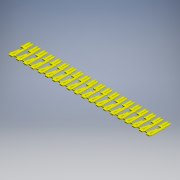
# Autodesk Inventor part: IDSD-20_pin
Saved by Autodesk Inventor 2017.3 (Build 213256000, 256)
## iProperties
Part Number: IDSD-20_pin
Material: Generic
Catalog Web Link: www.cadenas.de
Description: IDSS, IDSD Series - Pin-.100" Slim Body, IDC Ribbon Cable Assembly, Socket
Vendor: SAMTEC
Document SubType Name: Modeling
Designer: partserver
Manufacturer: SAMTEC
Mass: 0.0644285 g
Surface Area: 6.03509 cm^2
Volume: 0.0644285 cm^3
Density: 1 g/cm^3
Appearance: PSOLRGB-255-255-0
Category: PARTsolutions
Company: SAMTEC
Title: IDSD-20_pin
Author: Cadenas PARTsolutions
Comments: .100" Slim Body, IDC Ribbon Cable Assembly, Socket
PSOL_IDENT_0: {$CADENAS_DATA\23d-libs\samtec\modelling\idsd\parts\idsd_pin.prj},182 {VTYP=3D},{NB=IDSD-20_pin},{LI
PSOL_IDENT_1: NA=IDSD-20_pin},{NN=IDSS, IDSD Series - Pin},{DATE=12.08.2019 09:04:52},{GEOMDATE=04.12.2014 16:05:0
PSOL_IDENT_2: 0},{VERSION=},{LINEID=20},{WBVAR=POS},{WBNUMERIC=}  {NB=IDSD-20_pin},{LINA=IDSD-20_pin},{KT=DUMMY},{
PSOL_IDENT_3: PN=IDSD-20},{SERIES=IDSD},{POS=20},{POSNO=20},{A=2.05900000},{B=0.20},{C=0.10},{D=0.365}
NB: IDSD-20_pin
NN: IDSS, IDSD Series - Pin
NT: .100" Slim Body, IDC Ribbon Cable Assembly, Socket
NBSYN: $PN._pin
LINA: IDSD-20_pin
CATALOG: Samtec
SERIES: IDSD
POS: -20
B: 0.2
C: 0.1
SUPPLIER: SAMTEC
ARTICLENO: IDSD-20_pin
BOMINFO: IDSD-20_pin
CREATOR: CADENAS GmbH
Autodesk Inventor part; units mm, degrees
sketch "Sketch_4" plane through (0, 0, 0) normal (0, 0, 1) x (1, 0, 0)
  line L0 (-1.0795, 5.0292) -> (-0.8509, 4.5212)
  line L1 (-0.8509, 4.5212) -> (-0.8509, 0.635)
  line L2 (-0.8509, 0.635) -> (-0.4843, 0)
  line L3 (-0.4843, 0) -> (0.4843, 0)
  line L4 (0.4843, 0) -> (0.8509, 0.635)
  line L5 (0.8509, 0.635) -> (1.6891, 0.635)
  line L6 (1.6891, 0.635) -> (2.0557, 0)
  line L7 (2.0557, 0) -> (3.0243, 0)
  line L8 (3.0243, 0) -> (3.3909, 0.635)
  line L9 (3.3909, 0.635) -> (4.2291, 0.635)
  line L10 (4.2291, 0.635) -> (4.5957, 0)
  line L11 (4.5957, 0) -> (5.5643, 0)
  line L12 (5.5643, 0) -> (5.9309, 0.635)
  line L13 (5.9309, 0.635) -> (6.7691, 0.635)
  line L14 (6.7691, 0.635) -> (7.1357, 0)
  line L15 (7.1357, 0) -> (8.1043, 0)
  line L16 (8.1043, 0) -> (8.4709, 0.635)
  line L17 (8.4709, 0.635) -> (9.3091, 0.635)
  line L18 (9.3091, 0.635) -> (9.6757, 0)
  line L19 (9.6757, 0) -> (10.6443, 0)
  line L20 (10.6443, 0) -> (11.0109, 0.635)
  line L21 (11.0109, 0.635) -> (11.8491, 0.635)
  line L22 (11.8491, 0.635) -> (12.2157, 0)
  line L23 (12.2157, 0) -> (13.1843, 0)
  line L24 (13.1843, 0) -> (13.5509, 0.635)
  line L25 (13.5509, 0.635) -> (14.3891, 0.635)
  line L26 (14.3891, 0.635) -> (14.7557, 0)
  line L27 (14.7557, 0) -> (15.7243, 0)
  line L28 (15.7243, 0) -> (16.0909, 0.635)
  line L29 (16.0909, 0.635) -> (16.9291, 0.635)
  line L30 (16.9291, 0.635) -> (17.2957, 0)
  line L31 (17.2957, 0) -> (18.2643, 0)
  line L32 (18.2643, 0) -> (18.6309, 0.635)
  line L33 (18.6309, 0.635) -> (19.4691, 0.635)
  line L34 (19.4691, 0.635) -> (19.8357, 0)
  line L35 (19.8357, 0) -> (20.8043, 0)
  line L36 (20.8043, 0) -> (21.1709, 0.635)
  line L37 (21.1709, 0.635) -> (22.0091, 0.635)
  line L38 (22.0091, 0.635) -> (22.3757, 0)
  line L39 (22.3757, 0) -> (23.3443, 0)
  line L40 (23.3443, 0) -> (23.7109, 0.635)
  line L41 (23.7109, 0.635) -> (24.5491, 0.635)
  line L42 (24.5491, 0.635) -> (24.9157, 0)
  line L43 (24.9157, 0) -> (25.8843, 0)
  line L44 (25.8843, 0) -> (26.2509, 0.635)
  line L45 (26.2509, 0.635) -> (27.0891, 0.635)
  line L46 (27.0891, 0.635) -> (27.4557, 0)
  line L47 (27.4557, 0) -> (28.4243, 0)
  line L48 (28.4243, 0) -> (28.7909, 0.635)
  line L49 (28.7909, 0.635) -> (29.6291, 0.635)
  line L50 (29.6291, 0.635) -> (29.9957, 0)
  line L51 (29.9957, 0) -> (30.9643, 0)
  line L52 (30.9643, 0) -> (31.3309, 0.635)
  line L53 (31.3309, 0.635) -> (32.1691, 0.635)
  line L54 (32.1691, 0.635) -> (32.5357, 0)
  line L55 (32.5357, 0) -> (33.5043, 0)
  line L56 (33.5043, 0) -> (33.8709, 0.635)
  line L57 (33.8709, 0.635) -> (34.7091, 0.635)
  line L58 (34.7091, 0.635) -> (35.0757, 0)
  line L59 (35.0757, 0) -> (36.0443, 0)
  line L60 (36.0443, 0) -> (36.4109, 0.635)
  line L61 (36.4109, 0.635) -> (37.2491, 0.635)
  line L62 (37.2491, 0.635) -> (37.6157, 0)
  line L63 (37.6157, 0) -> (38.5843, 0)
  line L64 (38.5843, 0) -> (38.9509, 0.635)
  line L65 (38.9509, 0.635) -> (39.7891, 0.635)
  line L66 (39.7891, 0.635) -> (40.1557, 0)
  line L67 (40.1557, 0) -> (41.1243, 0)
  line L68 (41.1243, 0) -> (41.4909, 0.635)
  line L69 (41.4909, 0.635) -> (42.3291, 0.635)
  line L70 (42.3291, 0.635) -> (42.6957, 0)
  line L71 (42.6957, 0) -> (43.6643, 0)
  line L72 (43.6643, 0) -> (44.0309, 0.635)
  line L73 (44.0309, 0.635) -> (44.8691, 0.635)
  line L74 (44.8691, 0.635) -> (45.2357, 0)
  line L75 (45.2357, 0) -> (46.2043, 0)
  line L76 (46.2043, 0) -> (46.5709, 0.635)
  line L77 (46.5709, 0.635) -> (47.4091, 0.635)
  line L78 (47.4091, 0.635) -> (47.7757, 0)
  line L79 (47.7757, 0) -> (48.7443, 0)
  line L80 (48.7443, 0) -> (49.1109, 0.635)
  line L81 (49.1109, 0.635) -> (49.1109, 0.8128)
  line L82 (49.1109, 0.8128) -> (48.0695, 0.8128)
  line L83 (48.0695, 0.8128) -> (48.0695, 4.5212)
  line L84 (48.0695, 4.5212) -> (49.1109, 4.5212)
  line L85 (49.1109, 4.5212) -> (49.3395, 5.0292)
  line L86 (49.3395, 5.0292) -> (49.022, 5.0292)
  line L87 (49.022, 5.0292) -> (49.022, 6.8072)
  line L88 (49.022, 6.8072) -> (48.7934, 7.6962)
  line L89 (48.7934, 7.6962) -> (48.3616, 6.9483)
  line L90 (48.3616, 6.9483) -> (48.3616, 5.1562)
  line L91 (48.3616, 5.1562) -> (48.1584, 5.1562)
  line L92 (48.1584, 5.1562) -> (48.1584, 6.9483)
  line L93 (48.1584, 6.9483) -> (47.7266, 7.6962)
  line L94 (47.7266, 7.6962) -> (47.498, 6.8072)
  line L95 (47.498, 6.8072) -> (47.498, 5.0292)
  line L96 (47.498, 5.0292) -> (47.1805, 5.0292)
  line L97 (47.1805, 5.0292) -> (47.4091, 4.5212)
  line L98 (47.4091, 4.5212) -> (47.4091, 0.8128)
  line L99 (47.4091, 0.8128) -> (45.5295, 0.8128)
  line L100 (45.5295, 0.8128) -> (45.5295, 4.5212)
  line L101 (45.5295, 4.5212) -> (46.5709, 4.5212)
  line L102 (46.5709, 4.5212) -> (46.7995, 5.0292)
  line L103 (46.7995, 5.0292) -> (46.482, 5.0292)
  line L104 (46.482, 5.0292) -> (46.482, 6.8072)
  line L105 (46.482, 6.8072) -> (46.2534, 7.6962)
  line L106 (46.2534, 7.6962) -> (45.8216, 6.9483)
  line L107 (45.8216, 6.9483) -> (45.8216, 5.1562)
  line L108 (45.8216, 5.1562) -> (45.6184, 5.1562)
  line L109 (45.6184, 5.1562) -> (45.6184, 6.9483)
  line L110 (45.6184, 6.9483) -> (45.1866, 7.6962)
  line L111 (45.1866, 7.6962) -> (44.958, 6.8072)
  line L112 (44.958, 6.8072) -> (44.958, 5.0292)
  line L113 (44.958, 5.0292) -> (44.6405, 5.0292)
  line L114 (44.6405, 5.0292) -> (44.8691, 4.5212)
  line L115 (44.8691, 4.5212) -> (44.8691, 0.8128)
  line L116 (44.8691, 0.8128) -> (42.9895, 0.8128)
  line L117 (42.9895, 0.8128) -> (42.9895, 4.5212)
  line L118 (42.9895, 4.5212) -> (44.0309, 4.5212)
  line L119 (44.0309, 4.5212) -> (44.2595, 5.0292)
  line L120 (44.2595, 5.0292) -> (43.942, 5.0292)
  line L121 (43.942, 5.0292) -> (43.942, 6.8072)
  line L122 (43.942, 6.8072) -> (43.7134, 7.6962)
  line L123 (43.7134, 7.6962) -> (43.2816, 6.9483)
  line L124 (43.2816, 6.9483) -> (43.2816, 5.1562)
  line L125 (43.2816, 5.1562) -> (43.0784, 5.1562)
  line L126 (43.0784, 5.1562) -> (43.0784, 6.9483)
  line L127 (43.0784, 6.9483) -> (42.6466, 7.6962)
  line L128 (42.6466, 7.6962) -> (42.418, 6.8072)
  line L129 (42.418, 6.8072) -> (42.418, 5.0292)
  line L130 (42.418, 5.0292) -> (42.1005, 5.0292)
  line L131 (42.1005, 5.0292) -> (42.3291, 4.5212)
  line L132 (42.3291, 4.5212) -> (42.3291, 0.8128)
  line L133 (42.3291, 0.8128) -> (40.4495, 0.8128)
  line L134 (40.4495, 0.8128) -> (40.4495, 4.5212)
  line L135 (40.4495, 4.5212) -> (41.4909, 4.5212)
  line L136 (41.4909, 4.5212) -> (41.7195, 5.0292)
  line L137 (41.7195, 5.0292) -> (41.402, 5.0292)
  line L138 (41.402, 5.0292) -> (41.402, 6.8072)
  line L139 (41.402, 6.8072) -> (41.1734, 7.6962)
  line L140 (41.1734, 7.6962) -> (40.7416, 6.9483)
  line L141 (40.7416, 6.9483) -> (40.7416, 5.1562)
  line L142 (40.7416, 5.1562) -> (40.5384, 5.1562)
  line L143 (40.5384, 5.1562) -> (40.5384, 6.9483)
  line L144 (40.5384, 6.9483) -> (40.1066, 7.6962)
  line L145 (40.1066, 7.6962) -> (39.878, 6.8072)
  line L146 (39.878, 6.8072) -> (39.878, 5.0292)
  line L147 (39.878, 5.0292) -> (39.5605, 5.0292)
  line L148 (39.5605, 5.0292) -> (39.7891, 4.5212)
  line L149 (39.7891, 4.5212) -> (39.7891, 0.8128)
  line L150 (39.7891, 0.8128) -> (37.9095, 0.8128)
  line L151 (37.9095, 0.8128) -> (37.9095, 4.5212)
  line L152 (37.9095, 4.5212) -> (38.9509, 4.5212)
  line L153 (38.9509, 4.5212) -> (39.1795, 5.0292)
  line L154 (39.1795, 5.0292) -> (38.862, 5.0292)
  line L155 (38.862, 5.0292) -> (38.862, 6.8072)
  line L156 (38.862, 6.8072) -> (38.6334, 7.6962)
  line L157 (38.6334, 7.6962) -> (38.2016, 6.9483)
  line L158 (38.2016, 6.9483) -> (38.2016, 5.1562)
  line L159 (38.2016, 5.1562) -> (37.9984, 5.1562)
  line L160 (37.9984, 5.1562) -> (37.9984, 6.9483)
  line L161 (37.9984, 6.9483) -> (37.5666, 7.6962)
  line L162 (37.5666, 7.6962) -> (37.338, 6.8072)
  line L163 (37.338, 6.8072) -> (37.338, 5.0292)
  line L164 (37.338, 5.0292) -> (37.0205, 5.0292)
  line L165 (37.0205, 5.0292) -> (37.2491, 4.5212)
  line L166 (37.2491, 4.5212) -> (37.2491, 0.8128)
  line L167 (37.2491, 0.8128) -> (35.3695, 0.8128)
  line L168 (35.3695, 0.8128) -> (35.3695, 4.5212)
  line L169 (35.3695, 4.5212) -> (36.4109, 4.5212)
  line L170 (36.4109, 4.5212) -> (36.6395, 5.0292)
  line L171 (36.6395, 5.0292) -> (36.322, 5.0292)
  line L172 (36.322, 5.0292) -> (36.322, 6.8072)
  line L173 (36.322, 6.8072) -> (36.0934, 7.6962)
  line L174 (36.0934, 7.6962) -> (35.6616, 6.9483)
  line L175 (35.6616, 6.9483) -> (35.6616, 5.1562)
  line L176 (35.6616, 5.1562) -> (35.4584, 5.1562)
  line L177 (35.4584, 5.1562) -> (35.4584, 6.9483)
  line L178 (35.4584, 6.9483) -> (35.0266, 7.6962)
  line L179 (35.0266, 7.6962) -> (34.798, 6.8072)
  line L180 (34.798, 6.8072) -> (34.798, 5.0292)
  line L181 (34.798, 5.0292) -> (34.4805, 5.0292)
  line L182 (34.4805, 5.0292) -> (34.7091, 4.5212)
  line L183 (34.7091, 4.5212) -> (34.7091, 0.8128)
  line L184 (34.7091, 0.8128) -> (32.8295, 0.8128)
  line L185 (32.8295, 0.8128) -> (32.8295, 4.5212)
  line L186 (32.8295, 4.5212) -> (33.8709, 4.5212)
  line L187 (33.8709, 4.5212) -> (34.0995, 5.0292)
  line L188 (34.0995, 5.0292) -> (33.782, 5.0292)
  line L189 (33.782, 5.0292) -> (33.782, 6.8072)
  line L190 (33.782, 6.8072) -> (33.5534, 7.6962)
  line L191 (33.5534, 7.6962) -> (33.1216, 6.9483)
  line L192 (33.1216, 6.9483) -> (33.1216, 5.1562)
  line L193 (33.1216, 5.1562) -> (32.9184, 5.1562)
  line L194 (32.9184, 5.1562) -> (32.9184, 6.9483)
  line L195 (32.9184, 6.9483) -> (32.4866, 7.6962)
  line L196 (32.4866, 7.6962) -> (32.258, 6.8072)
  line L197 (32.258, 6.8072) -> (32.258, 5.0292)
  line L198 (32.258, 5.0292) -> (31.9405, 5.0292)
  line L199 (31.9405, 5.0292) -> (32.1691, 4.5212)
  line L200 (32.1691, 4.5212) -> (32.1691, 0.8128)
  line L201 (32.1691, 0.8128) -> (30.2895, 0.8128)
  line L202 (30.2895, 0.8128) -> (30.2895, 4.5212)
  line L203 (30.2895, 4.5212) -> (31.3309, 4.5212)
  line L204 (31.3309, 4.5212) -> (31.5595, 5.0292)
  line L205 (31.5595, 5.0292) -> (31.242, 5.0292)
  line L206 (31.242, 5.0292) -> (31.242, 6.8072)
  line L207 (31.242, 6.8072) -> (31.0134, 7.6962)
  line L208 (31.0134, 7.6962) -> (30.5816, 6.9483)
  line L209 (30.5816, 6.9483) -> (30.5816, 5.1562)
  line L210 (30.5816, 5.1562) -> (30.3784, 5.1562)
  line L211 (30.3784, 5.1562) -> (30.3784, 6.9483)
  line L212 (30.3784, 6.9483) -> (29.9466, 7.6962)
  line L213 (29.9466, 7.6962) -> (29.718, 6.8072)
  line L214 (29.718, 6.8072) -> (29.718, 5.0292)
  line L215 (29.718, 5.0292) -> (29.4005, 5.0292)
  line L216 (29.4005, 5.0292) -> (29.6291, 4.5212)
  line L217 (29.6291, 4.5212) -> (29.6291, 0.8128)
  line L218 (29.6291, 0.8128) -> (27.7495, 0.8128)
  line L219 (27.7495, 0.8128) -> (27.7495, 4.5212)
  line L220 (27.7495, 4.5212) -> (28.7909, 4.5212)
  line L221 (28.7909, 4.5212) -> (29.0195, 5.0292)
  line L222 (29.0195, 5.0292) -> (28.702, 5.0292)
  line L223 (28.702, 5.0292) -> (28.702, 6.8072)
  line L224 (28.702, 6.8072) -> (28.4734, 7.6962)
  line L225 (28.4734, 7.6962) -> (28.0416, 6.9483)
  line L226 (28.0416, 6.9483) -> (28.0416, 5.1562)
  line L227 (28.0416, 5.1562) -> (27.8384, 5.1562)
  line L228 (27.8384, 5.1562) -> (27.8384, 6.9483)
  line L229 (27.8384, 6.9483) -> (27.4066, 7.6962)
  line L230 (27.4066, 7.6962) -> (27.178, 6.8072)
  line L231 (27.178, 6.8072) -> (27.178, 5.0292)
  line L232 (27.178, 5.0292) -> (26.8605, 5.0292)
  line L233 (26.8605, 5.0292) -> (27.0891, 4.5212)
  line L234 (27.0891, 4.5212) -> (27.0891, 0.8128)
  line L235 (27.0891, 0.8128) -> (25.2095, 0.8128)
  line L236 (25.2095, 0.8128) -> (25.2095, 4.5212)
  line L237 (25.2095, 4.5212) -> (26.2509, 4.5212)
  line L238 (26.2509, 4.5212) -> (26.4795, 5.0292)
  line L239 (26.4795, 5.0292) -> (26.162, 5.0292)
  line L240 (26.162, 5.0292) -> (26.162, 6.8072)
  line L241 (26.162, 6.8072) -> (25.9334, 7.6962)
  line L242 (25.9334, 7.6962) -> (25.5016, 6.9483)
  line L243 (25.5016, 6.9483) -> (25.5016, 5.1562)
  line L244 (25.5016, 5.1562) -> (25.2984, 5.1562)
  line L245 (25.2984, 5.1562) -> (25.2984, 6.9483)
  line L246 (25.2984, 6.9483) -> (24.8666, 7.6962)
  line L247 (24.8666, 7.6962) -> (24.638, 6.8072)
  line L248 (24.638, 6.8072) -> (24.638, 5.0292)
  line L249 (24.638, 5.0292) -> (24.3205, 5.0292)
  line L250 (24.3205, 5.0292) -> (24.5491, 4.5212)
  line L251 (24.5491, 4.5212) -> (24.5491, 0.8128)
  line L252 (24.5491, 0.8128) -> (22.6695, 0.8128)
  line L253 (22.6695, 0.8128) -> (22.6695, 4.5212)
  line L254 (22.6695, 4.5212) -> (23.7109, 4.5212)
  line L255 (23.7109, 4.5212) -> (23.9395, 5.0292)
  line L256 (23.9395, 5.0292) -> (23.622, 5.0292)
  line L257 (23.622, 5.0292) -> (23.622, 6.8072)
  line L258 (23.622, 6.8072) -> (23.3934, 7.6962)
  line L259 (23.3934, 7.6962) -> (22.9616, 6.9483)
  line L260 (22.9616, 6.9483) -> (22.9616, 5.1562)
  line L261 (22.9616, 5.1562) -> (22.7584, 5.1562)
  line L262 (22.7584, 5.1562) -> (22.7584, 6.9483)
  line L263 (22.7584, 6.9483) -> (22.3266, 7.6962)
  line L264 (22.3266, 7.6962) -> (22.098, 6.8072)
  line L265 (22.098, 6.8072) -> (22.098, 5.0292)
  line L266 (22.098, 5.0292) -> (21.7805, 5.0292)
  line L267 (21.7805, 5.0292) -> (22.0091, 4.5212)
  line L268 (22.0091, 4.5212) -> (22.0091, 0.8128)
  line L269 (22.0091, 0.8128) -> (20.1295, 0.8128)
  line L270 (20.1295, 0.8128) -> (20.1295, 4.5212)
  line L271 (20.1295, 4.5212) -> (21.1709, 4.5212)
  line L272 (21.1709, 4.5212) -> (21.3995, 5.0292)
  line L273 (21.3995, 5.0292) -> (21.082, 5.0292)
  line L274 (21.082, 5.0292) -> (21.082, 6.8072)
  line L275 (21.082, 6.8072) -> (20.8534, 7.6962)
  line L276 (20.8534, 7.6962) -> (20.4216, 6.9483)
  line L277 (20.4216, 6.9483) -> (20.4216, 5.1562)
  line L278 (20.4216, 5.1562) -> (20.2184, 5.1562)
  line L279 (20.2184, 5.1562) -> (20.2184, 6.9483)
  line L280 (20.2184, 6.9483) -> (19.7866, 7.6962)
  line L281 (19.7866, 7.6962) -> (19.558, 6.8072)
  line L282 (19.558, 6.8072) -> (19.558, 5.0292)
  line L283 (19.558, 5.0292) -> (19.2405, 5.0292)
  line L284 (19.2405, 5.0292) -> (19.4691, 4.5212)
  line L285 (19.4691, 4.5212) -> (19.4691, 0.8128)
  line L286 (19.4691, 0.8128) -> (17.5895, 0.8128)
  line L287 (17.5895, 0.8128) -> (17.5895, 4.5212)
  line L288 (17.5895, 4.5212) -> (18.6309, 4.5212)
  line L289 (18.6309, 4.5212) -> (18.8595, 5.0292)
  line L290 (18.8595, 5.0292) -> (18.542, 5.0292)
  line L291 (18.542, 5.0292) -> (18.542, 6.8072)
  line L292 (18.542, 6.8072) -> (18.3134, 7.6962)
  line L293 (18.3134, 7.6962) -> (17.8816, 6.9483)
  line L294 (17.8816, 6.9483) -> (17.8816, 5.1562)
  line L295 (17.8816, 5.1562) -> (17.6784, 5.1562)
  line L296 (17.6784, 5.1562) -> (17.6784, 6.9483)
  line L297 (17.6784, 6.9483) -> (17.2466, 7.6962)
  line L298 (17.2466, 7.6962) -> (17.018, 6.8072)
  line L299 (17.018, 6.8072) -> (17.018, 5.0292)
  line L300 (17.018, 5.0292) -> (16.7005, 5.0292)
  line L301 (16.7005, 5.0292) -> (16.9291, 4.5212)
  line L302 (16.9291, 4.5212) -> (16.9291, 0.8128)
  line L303 (16.9291, 0.8128) -> (15.0495, 0.8128)
  line L304 (15.0495, 0.8128) -> (15.0495, 4.5212)
  line L305 (15.0495, 4.5212) -> (16.0909, 4.5212)
  line L306 (16.0909, 4.5212) -> (16.3195, 5.0292)
  line L307 (16.3195, 5.0292) -> (16.002, 5.0292)
  line L308 (16.002, 5.0292) -> (16.002, 6.8072)
  line L309 (16.002, 6.8072) -> (15.7734, 7.6962)
  line L310 (15.7734, 7.6962) -> (15.3416, 6.9483)
  line L311 (15.3416, 6.9483) -> (15.3416, 5.1562)
  line L312 (15.3416, 5.1562) -> (15.1384, 5.1562)
  line L313 (15.1384, 5.1562) -> (15.1384, 6.9483)
  line L314 (15.1384, 6.9483) -> (14.7066, 7.6962)
  line L315 (14.7066, 7.6962) -> (14.478, 6.8072)
  line L316 (14.478, 6.8072) -> (14.478, 5.0292)
  line L317 (14.478, 5.0292) -> (14.1605, 5.0292)
  line L318 (14.1605, 5.0292) -> (14.3891, 4.5212)
  line L319 (14.3891, 4.5212) -> (14.3891, 0.8128)
  line L320 (14.3891, 0.8128) -> (12.5095, 0.8128)
  line L321 (12.5095, 0.8128) -> (12.5095, 4.5212)
  line L322 (12.5095, 4.5212) -> (13.5509, 4.5212)
  line L323 (13.5509, 4.5212) -> (13.7795, 5.0292)
  line L324 (13.7795, 5.0292) -> (13.462, 5.0292)
  line L325 (13.462, 5.0292) -> (13.462, 6.8072)
  line L326 (13.462, 6.8072) -> (13.2334, 7.6962)
  line L327 (13.2334, 7.6962) -> (12.8016, 6.9483)
  line L328 (12.8016, 6.9483) -> (12.8016, 5.1562)
  line L329 (12.8016, 5.1562) -> (12.5984, 5.1562)
  line L330 (12.5984, 5.1562) -> (12.5984, 6.9483)
  line L331 (12.5984, 6.9483) -> (12.1666, 7.6962)
  line L332 (12.1666, 7.6962) -> (11.938, 6.8072)
  line L333 (11.938, 6.8072) -> (11.938, 5.0292)
  line L334 (11.938, 5.0292) -> (11.6205, 5.0292)
  line L335 (11.6205, 5.0292) -> (11.8491, 4.5212)
  line L336 (11.8491, 4.5212) -> (11.8491, 0.8128)
  line L337 (11.8491, 0.8128) -> (9.9695, 0.8128)
  line L338 (9.9695, 0.8128) -> (9.9695, 4.5212)
  line L339 (9.9695, 4.5212) -> (11.0109, 4.5212)
  line L340 (11.0109, 4.5212) -> (11.2395, 5.0292)
  line L341 (11.2395, 5.0292) -> (10.922, 5.0292)
  line L342 (10.922, 5.0292) -> (10.922, 6.8072)
  line L343 (10.922, 6.8072) -> (10.6934, 7.6962)
  line L344 (10.6934, 7.6962) -> (10.2616, 6.9483)
  line L345 (10.2616, 6.9483) -> (10.2616, 5.1562)
  line L346 (10.2616, 5.1562) -> (10.0584, 5.1562)
  line L347 (10.0584, 5.1562) -> (10.0584, 6.9483)
  line L348 (10.0584, 6.9483) -> (9.6266, 7.6962)
  line L349 (9.6266, 7.6962) -> (9.398, 6.8072)
  line L350 (9.398, 6.8072) -> (9.398, 5.0292)
  line L351 (9.398, 5.0292) -> (9.0805, 5.0292)
  line L352 (9.0805, 5.0292) -> (9.3091, 4.5212)
  line L353 (9.3091, 4.5212) -> (9.3091, 0.8128)
  line L354 (9.3091, 0.8128) -> (7.4295, 0.8128)
  line L355 (7.4295, 0.8128) -> (7.4295, 4.5212)
  line L356 (7.4295, 4.5212) -> (8.4709, 4.5212)
  line L357 (8.4709, 4.5212) -> (8.6995, 5.0292)
  line L358 (8.6995, 5.0292) -> (8.382, 5.0292)
  line L359 (8.382, 5.0292) -> (8.382, 6.8072)
  line L360 (8.382, 6.8072) -> (8.1534, 7.6962)
  line L361 (8.1534, 7.6962) -> (7.7216, 6.9483)
  line L362 (7.7216, 6.9483) -> (7.7216, 5.1562)
  line L363 (7.7216, 5.1562) -> (7.5184, 5.1562)
  line L364 (7.5184, 5.1562) -> (7.5184, 6.9483)
  line L365 (7.5184, 6.9483) -> (7.0866, 7.6962)
  line L366 (7.0866, 7.6962) -> (6.858, 6.8072)
  line L367 (6.858, 6.8072) -> (6.858, 5.0292)
  line L368 (6.858, 5.0292) -> (6.5405, 5.0292)
  line L369 (6.5405, 5.0292) -> (6.7691, 4.5212)
  line L370 (6.7691, 4.5212) -> (6.7691, 0.8128)
  line L371 (6.7691, 0.8128) -> (4.8895, 0.8128)
  line L372 (4.8895, 0.8128) -> (4.8895, 4.5212)
  line L373 (4.8895, 4.5212) -> (5.9309, 4.5212)
  line L374 (5.9309, 4.5212) -> (6.1595, 5.0292)
  line L375 (6.1595, 5.0292) -> (5.842, 5.0292)
  line L376 (5.842, 5.0292) -> (5.842, 6.8072)
  line L377 (5.842, 6.8072) -> (5.6134, 7.6962)
  line L378 (5.6134, 7.6962) -> (5.1816, 6.9483)
  line L379 (5.1816, 6.9483) -> (5.1816, 5.1562)
  line L380 (5.1816, 5.1562) -> (4.9784, 5.1562)
  line L381 (4.9784, 5.1562) -> (4.9784, 6.9483)
  line L382 (4.9784, 6.9483) -> (4.5466, 7.6962)
  line L383 (4.5466, 7.6962) -> (4.318, 6.8072)
  line L384 (4.318, 6.8072) -> (4.318, 5.0292)
  line L385 (4.318, 5.0292) -> (4.0005, 5.0292)
  line L386 (4.0005, 5.0292) -> (4.2291, 4.5212)
  line L387 (4.2291, 4.5212) -> (4.2291, 0.8128)
  line L388 (4.2291, 0.8128) -> (2.3495, 0.8128)
  line L389 (2.3495, 0.8128) -> (2.3495, 4.5212)
  line L390 (2.3495, 4.5212) -> (3.3909, 4.5212)
  line L391 (3.3909, 4.5212) -> (3.6195, 5.0292)
  line L392 (3.6195, 5.0292) -> (3.302, 5.0292)
  line L393 (3.302, 5.0292) -> (3.302, 6.8072)
  line L394 (3.302, 6.8072) -> (3.0734, 7.6962)
  line L395 (3.0734, 7.6962) -> (2.6416, 6.9483)
  line L396 (2.6416, 6.9483) -> (2.6416, 5.1562)
  line L397 (2.6416, 5.1562) -> (2.4384, 5.1562)
  line L398 (2.4384, 5.1562) -> (2.4384, 6.9483)
  line L399 (2.4384, 6.9483) -> (2.0066, 7.6962)
  line L400 (2.0066, 7.6962) -> (1.778, 6.8072)
  line L401 (1.778, 6.8072) -> (1.778, 5.0292)
  line L402 (1.778, 5.0292) -> (1.4605, 5.0292)
  line L403 (1.4605, 5.0292) -> (1.6891, 4.5212)
  line L404 (1.6891, 4.5212) -> (1.6891, 0.8128)
  line L405 (1.6891, 0.8128) -> (-0.1905, 0.8128)
  line L406 (-0.1905, 0.8128) -> (-0.1905, 4.5212)
  line L407 (-0.1905, 4.5212) -> (0.8509, 4.5212)
  line L408 (0.8509, 4.5212) -> (1.0795, 5.0292)
  line L409 (1.0795, 5.0292) -> (0.762, 5.0292)
  line L410 (0.762, 5.0292) -> (0.762, 6.8072)
  line L411 (0.762, 6.8072) -> (0.5334, 7.6962)
  line L412 (0.5334, 7.6962) -> (0.1016, 6.9483)
  line L413 (0.1016, 6.9483) -> (0.1016, 5.1562)
  line L414 (0.1016, 5.1562) -> (-0.1016, 5.1562)
  line L415 (-0.1016, 5.1562) -> (-0.1016, 6.9483)
  line L416 (-0.1016, 6.9483) -> (-0.5334, 7.6962)
  line L417 (-0.5334, 7.6962) -> (-0.762, 6.8072)
  line L418 (-0.762, 6.8072) -> (-0.762, 5.0292)
  line L419 (-0.762, 5.0292) -> (-1.0795, 5.0292)
  constraints: 840 end point
extrude "Extrusion1" add sketch "Sketch_4" against normal blind 0.3302
sketch "Sketch_2" plane through (0.8509, 0, 0) normal (1, 0, 0) x (0, 0, -1)
  line L0 (-0.4826, 3.2004) -> (0, 0.8763)
  line L1 (0, 0.8763) -> (0, 0.8128)
  line L2 (0, 0.8128) -> (0.3302, 0.8128)
  line L3 (0.3302, 0.8128) -> (0.3302, 0.9102)
  line L4 (0.3302, 0.9102) -> (-0.1524, 3.2343)
  line L5 (-0.1524, 3.2343) -> (-0.1524, 3.81)
  line L6 (-0.1524, 3.81) -> (-0.4826, 3.81)
  line L7 (-0.4826, 3.81) -> (-0.4826, 3.2004)
  constraints: 16 end point
extrude "Extrusion2" add sketch "Sketch_2" against normal blind 0.6604
pattern_linear "Rectangular Pattern1" count 20 spacing 2.54 along (1, 0, 0) of "Extrusion2"
ref_plane "pin_XY" through (0.635, 0, 0.4318) normal (0, 1, 0) x (1, 0, 0)
ref_plane "pin_YZ" through (0.635, 0, 0.4318) normal (1, 0, 0) x (0, 0, -1)
ref_plane "pin_ZX" through (0.635, 0, 0.4318) normal (0, 0, -1) x (0, 1, 0)
ref_plane "pin_reverse_XY" through (0.635, 0, 0.4318) normal (0, -1, 0) x (1, 0, 0)
ref_plane "pin_reverse_YZ" through (0.635, 0, 0.4318) normal (1, 0, 0) x (0, 0, 1)
ref_plane "pin_reverse_ZX" through (0.635, 0, 0.4318) normal (0, 0, 1) x (0, -1, 0)
body "Solid1"
